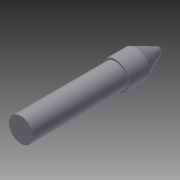
# Autodesk Inventor part: soldering_lead_tube
Saved by Autodesk Inventor 2013 (Build 170138000, 138)
## iProperties
Created: 2013-03-19
Part Number: soldering_lead_tube
Material: Generic
Document SubType Name: Modeling
Designer: Mahisorn
Density: 1 g/cm^3
Author: Mahisorn
Autodesk Inventor part; units mm, degrees
ref_plane "YZ Plane" through (0, 0, 0) normal (1, 0, 0) x (0, 1, 0)
ref_plane "XZ Plane" through (0, 0, 0) normal (0, 1, 0) x (-1, 0, 0)
ref_plane "XY Plane" through (0, 0, 0) normal (0, 0, 1) x (1, 0, 0)
sketch "Sketch1" plane through (0, 0, 0) normal (0, 0, 1) x (1, 0, 0)
  line L0 (0, 0) -> (-8.25, 0)
  line L1 (-8.25, 0) -> (-8.25, 65)
  line L2 (-8.25, 65) -> (-9.5, 65)
  line L3 (-9.5, 65) -> (-9.5, 79)
  line L4 (0, 0) -> (0, 95)
  line L5 (0, 95) -> (-2, 95)
  line L6 (-2, 95) -> (-9.5, 79)
  dimension "d0" = 8.25
  dimension "d1" = 65
  dimension "d2" = 1.25
  dimension "d3" = 14
  dimension "d4" = 95
  dimension "d5" = 2
  constraints: 14 end point, 4 perpendicular, 1 horizontal, 1 parallel
  measures "d0" distance of L0.start L0.end
  measures "d1" distance of L0.end L1.end
  measures "d2" distance of L1.end L2.end
  measures "d3" distance of L2.end L3.end
  measures "d4" distance of L0.start L4.end
  measures "d5" distance of L4.end L5.end
revolve "Revolution1" add sketch "Sketch1" angle 360 about axis through (0, 0, 0) along (0, 1, 0)
body "Solid1"
